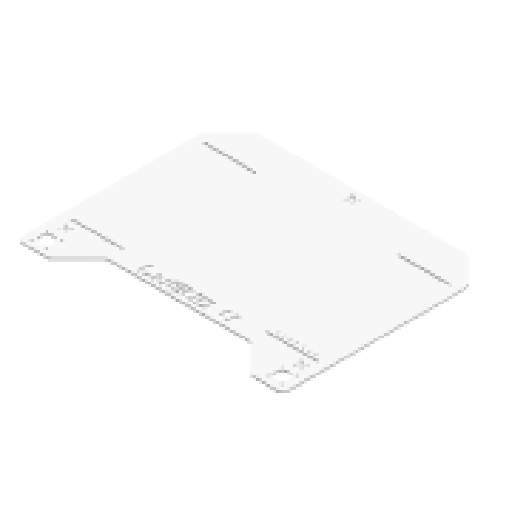
# Autodesk Inventor part: Z Axis Base
Saved by Autodesk Inventor 2023.2 (Build 272271000, 271)
## iProperties
Created: 2023-02-02
Part Number: Z Axis Base
Material: Aluminum 6061
Document SubType Name: Modeling
Designer: remop
Density: 2.7 g/cm^3
Appearance: Aluminum - Dark
Author: remop
Autodesk Inventor part; units mm, degrees
ref_plane "YZ Plane" through (0, 0, 0) normal (1, 0, 0) x (0, 1, 0)
ref_plane "XZ Plane" through (0, 0, 0) normal (0, 1, 0) x (-1, 0, 0)
ref_plane "XY Plane" through (0, 0, 0) normal (0, 0, 1) x (1, 0, 0)
sketch "Sketch1" plane through (0, 0, 0) normal (0, 1, 0) x (-1, 0, 0)
  circle A0 centre (158.2314, 130.3812) radius 11.25 projected
  circle A1 centre (158.2314, 160.3812) radius 6 projected
  circle A2 centre (-213.7686, 130.3812) radius 11.25 projected
  circle A3 centre (-213.7686, 160.3812) radius 6 projected
  circle A4 centre (-27.7686, -135.6188) radius 11 projected
  circle A5 centre (125.7314, 112.8812) radius 1.75
  circle A6 centre (125.7314, -96.1188) radius 1.75
  circle A7 centre (-181.2686, -96.1188) radius 1.75
  circle A8 centre (-181.2686, 112.8812) radius 1.75
  line L0 (222.2314, 188.3812) -> (-277.7686, 188.3812) projected
  line L1 (222.2314, -171.6188) -> (-277.7686, -171.6188) projected
  line L2 (182.2314, 183.3812) -> (132.2314, 183.3812)
  line L3 (132.2314, 183.3812) -> (86.7314, 137.8812)
  line L4 (86.7314, 137.8812) -> (-142.2686, 137.8812)
  line L5 (-142.2686, 137.8812) -> (-187.7686, 183.3812)
  line L6 (-187.7686, 183.3812) -> (-237.7686, 183.3812)
  line L7 (-237.7686, 183.3812) -> (-237.7686, -151.6188)
  line L8 (-237.7686, -151.6188) -> (182.2314, -151.6188)
  line L9 (182.2314, -151.6188) -> (182.2314, 183.3812)
  line L10 (222.2314, -171.6188) -> (222.2314, 188.3812) projected
  line L11 (-277.7686, 188.3812) -> (-277.7686, -171.6188) projected
  circle A9 centre (-213.7686, 160.3812) radius 11.5
  circle A10 centre (-225.2686, 171.8812) radius 2.1
  circle A11 centre (-202.2686, 171.8812) radius 2.1
  circle A12 centre (-202.2686, 148.8812) radius 2.1
  circle A13 centre (-225.2686, 148.8812) radius 2.1
  circle A14 centre (158.2314, 160.3812) radius 11.5
  circle A15 centre (146.7314, 171.8812) radius 2.1
  circle A16 centre (169.7314, 171.8812) radius 2.1
  circle A17 centre (169.7314, 148.8812) radius 2.1
  circle A18 centre (146.7314, 148.8812) radius 2.1
  circle A19 centre (-213.7686, 130.3812) radius 4.5
  circle A20 centre (-219.2686, 124.8812) radius 1.6
  circle A21 centre (-219.2686, 135.8812) radius 1.6
  circle A22 centre (-208.2686, 135.8812) radius 1.6
  circle A23 centre (-208.2686, 124.8812) radius 1.6
  circle A24 centre (158.2314, 130.3812) radius 4.5
  circle A25 centre (152.7314, 135.8812) radius 1.6
  circle A26 centre (163.7314, 135.8812) radius 1.6
  circle A27 centre (163.7314, 124.8812) radius 1.6
  circle A28 centre (152.7314, 124.8812) radius 1.6
  circle A29 centre (-27.7686, -135.6188) radius 4.5
  circle A30 centre (-33.2686, -130.1188) radius 1.6
  circle A31 centre (-22.2686, -130.1188) radius 1.6
  circle A32 centre (-22.2686, -141.1188) radius 1.6
  circle A33 centre (-33.2686, -141.1188) radius 1.6
  point P0 (0, 0)
  point P1 (157.2314, 183.3812)
  dimension "d0" = 307
  dimension "d1" = 209
  dimension "d2" = 3.5
  dimension "d3" = 153.5
  dimension "d4" = 360
  dimension "d5" = 75.5
  dimension "d6" = 5
  dimension "d7" = 40
  dimension "d8" = 20
  dimension "d9" = 40
  dimension "d10" = 5
  dimension "d12" = 45
  dimension "d13" = 50
  dimension "d14" = 45
  dimension "d15" = 25
  dimension "d18" = 23
  dimension "d19" = 11.5
  dimension "d20" = 11.5
  dimension "d21" = 11.5
  dimension "d22" = 11.5
  dimension "d23" = 4.2
  dimension "d24" = 11.5
  dimension "d25" = 11.5
  dimension "d26" = 11.5
  dimension "d27" = 11.5
  dimension "d28" = 9
  dimension "d29" = 5.5
  dimension "d30" = 5.5
  dimension "d31" = 5.5
  dimension "d32" = 5.5
  dimension "d33" = 3.2
  dimension "d35" = 5.5
  dimension "d36" = 5.5
  dimension "d37" = 5.5
  dimension "d39" = 5.5
  dimension "d40" = 5.5
  dimension "d41" = 5.5
  dimension "d42" = 5.5
  dimension "d43" = 5.5
  constraints: 29 centre point, 24 equal radius, 16 end point, 12 horizontal alignment, 12 vertical alignment, 5 coincident, 3 parallel, 1 collinear, 1 horizontal, 1 midpoint, 1 perpendicular
  measures "d0" distance of A8.centre A5.centre
  measures "d1" distance of A6.centre A5.centre
  measures "d2" diameter of A5
  measures "d3" horizontal distance of A6.centre A4.centre
  measures "d4" distance between parallel lines of L1 L0
  measures "d5" distance from line of L1 A7.centre
  measures "d6" distance between parallel lines of L0 L6
  measures "d7" distance between parallel lines of L11 L7
  measures "d8" distance between parallel lines of L1 L8
  measures "d9" distance between parallel lines of L10 L9
  measures "d10" distance from line of L0 point (157.231, 183.381)
  measures "d12" angle of L2 L3
  measures "d13" distance of L2.start L2.end
  measures "d14" angle of L6 L5
  measures "d15" distance from line of A5.centre L4
  measures "d18" diameter of A9
  measures "d19" horizontal distance of A3.centre A10.centre
  measures "d20" horizontal distance of A3.centre A11.centre
  measures "d21" horizontal distance of A10.centre A9.centre
  measures "d22" horizontal distance of A13.centre A3.centre
  measures "d23" diameter of A13
  measures "d24" horizontal distance of A15.centre A1.centre
  measures "d25" horizontal distance of A18.centre A1.centre
  measures "d26" horizontal distance of A1.centre A18.centre
  measures "d27" horizontal distance of A17.centre A14.centre
  measures "d28" diameter of A19
  measures "d29" horizontal distance of A21.centre A2.centre
  measures "d30" horizontal distance of A19.centre A21.centre
  measures "d31" horizontal distance of A22.centre A2.centre
  measures "d32" horizontal distance of A20.centre A2.centre
  measures "d33" diameter of A20
  measures "d35" horizontal distance of A25.centre A0.centre
  measures "d36" horizontal distance of A25.centre A0.centre
  measures "d37" horizontal distance of A0.centre A26.centre
  measures "d39" horizontal distance of A0.centre A28.centre
  measures "d40" horizontal distance of A31.centre A29.centre
  measures "d41" horizontal distance of A30.centre A4.centre
  measures "d42" horizontal distance of A31.centre A29.centre
  measures "d43" horizontal distance of A32.centre A29.centre
extrude "Extrusion1" add sketch "Sketch1" along normal blind 3 contours A0 | A2 | A4 | L9 L8 L7 L6 L5 L4 L3 L2
sketch "Sketch2" plane through (0, 3, 0) normal (0, 1, 0) x (1, 0, 0)
  line L0 (-132.2314, -183.3812) -> (-86.7314, -137.8812) projected
  line L1 (-86.7314, -137.8812) -> (142.2686, -137.8812) projected
  line L2 (142.2686, -137.8812) -> (187.7686, -183.3812) projected
  line L3 (187.7686, -183.3812) -> (237.7686, -183.3812) projected
  line L4 (237.7686, -183.3812) -> (237.7686, 151.6188) projected
  line L5 (237.7686, 151.6188) -> (-182.2314, 151.6188) projected
  line L6 (-182.2314, 151.6188) -> (-182.2314, -183.3812) projected
  line L7 (-182.2314, -183.3812) -> (-132.2314, -183.3812) projected
  circle A0 centre (-158.2314, -130.3812) radius 4.5 projected
  circle A1 centre (-152.7314, -135.8812) radius 1.6 projected
  circle A2 centre (-163.7314, -135.8812) radius 1.6 projected
  circle A3 centre (-163.7314, -124.8812) radius 1.6 projected
  circle A4 centre (-152.7314, -124.8812) radius 1.6 projected
  circle A5 centre (213.7686, -130.3812) radius 4.5 projected
  circle A6 centre (219.2686, -124.8812) radius 1.6 projected
  circle A7 centre (219.2686, -135.8812) radius 1.6 projected
  circle A8 centre (208.2686, -135.8812) radius 1.6 projected
  circle A9 centre (208.2686, -124.8812) radius 1.6 projected
  circle A10 centre (27.7686, 135.6188) radius 4.5 projected
  circle A11 centre (33.2686, 130.1188) radius 1.6 projected
  circle A12 centre (22.2686, 130.1188) radius 1.6 projected
  circle A13 centre (22.2686, 141.1188) radius 1.6 projected
  circle A14 centre (33.2686, 141.1188) radius 1.6 projected
  circle A15 centre (-125.7314, -112.8812) radius 1.75 projected
  circle A16 centre (-125.7314, 96.1188) radius 1.75 projected
  circle A17 centre (181.2686, 96.1188) radius 1.75 projected
  circle A18 centre (181.2686, -112.8812) radius 1.75 projected
  circle A19 centre (-146.7314, -148.8812) radius 2.1 projected
  circle A20 centre (-169.7314, -148.8812) radius 2.1 projected
  circle A21 centre (-169.7314, -171.8812) radius 2.1 projected
  circle A22 centre (-146.7314, -171.8812) radius 2.1 projected
  circle A23 centre (-158.2314, -160.3812) radius 11.5 projected
  circle A24 centre (225.2686, -148.8812) radius 2.1 projected
  circle A25 centre (202.2686, -148.8812) radius 2.1 projected
  circle A26 centre (202.2686, -171.8812) radius 2.1 projected
  circle A27 centre (225.2686, -171.8812) radius 2.1 projected
  circle A28 centre (213.7686, -160.3812) radius 11.5 projected
  line L8 (-71.2064, -116.1262) -> (126.7436, -116.1262) construction
  line L9 (126.7436, -116.1262) -> (126.7436, -129.6362) construction
  line L10 (126.7436, -129.6362) -> (-71.2064, -129.6362) construction
  line L11 (-71.2064, -129.6362) -> (-71.2064, -116.1262) construction
  line L12 (-41.9641, -132.872) -> (-44.5632, -130.2729)
  line L13 (-44.5632, -130.2729) -> (-44.5632, -112.872)
  line L14 (-44.5632, -112.872) -> (-37.5955, -112.872)
  line L15 (-37.5955, -112.872) -> (-37.5955, -132.872)
  line L16 (-37.5955, -132.872) -> (-41.9641, -132.872)
  line L17 (-36.7844, -132.872) -> (-36.7844, -126.9549)
  line L18 (-36.7844, -126.9549) -> (-23.66, -126.9549)
  line L19 (-23.66, -126.9549) -> (-23.66, -132.872)
  line L20 (-23.66, -132.872) -> (-36.7844, -132.872)
  line L21 (-9.3743, -132.8536) -> (-19.3282, -132.8536)
  line L22 (-19.3282, -132.8536) -> (-22.554, -129.6277)
  line L23 (-22.554, -129.6277) -> (-22.554, -118.4388)
  line L24 (-22.554, -118.4388) -> (-15.4941, -118.4388)
  line L25 (-15.4941, -118.4388) -> (-15.4941, -126.9365)
  line L26 (-15.4941, -126.9365) -> (-9.3743, -126.9365)
  line L27 (-9.3743, -126.9365) -> (-9.3743, -132.8536)
  line L28 (-1.5402, -132.8536) -> (-8.6001, -132.8536)
  line L29 (-8.6001, -132.8536) -> (-8.6001, -118.4388)
  line L30 (-8.6001, -118.4388) -> (-1.5402, -118.4388)
  line L31 (-1.5402, -118.4388) -> (-1.5402, -132.8536)
  line L32 (6.5889, -132.872) -> (2.1649, -132.872)
  line L33 (2.1649, -132.872) -> (-0.4342, -130.2729)
  line L34 (-0.4342, -130.2729) -> (-0.4342, -115.4711)
  line L35 (-0.4342, -115.4711) -> (2.1649, -112.872)
  line L36 (2.1649, -112.872) -> (6.5889, -112.872)
  line L37 (6.5889, -112.872) -> (6.5889, -132.872)
  line L38 (20.5797, -119.0471) -> (7.3999, -119.0471)
  line L39 (7.3999, -119.0471) -> (7.3999, -112.872)
  line L40 (7.3999, -112.872) -> (20.5797, -112.872)
  line L41 (20.5797, -112.872) -> (20.5797, -119.0471)
  line L42 (20.5797, -132.872) -> (7.3999, -132.872)
  line L43 (7.3999, -132.872) -> (7.3999, -126.9549)
  line L44 (7.3999, -126.9549) -> (20.5797, -126.9549)
  line L45 (20.5797, -126.9549) -> (20.5797, -132.872)
  line L46 (20.5797, -124.7061) -> (7.3999, -124.7061)
  line L47 (7.3999, -124.7061) -> (7.3999, -119.8582)
  line L48 (7.3999, -119.8582) -> (20.5797, -119.8582)
  line L49 (20.5797, -119.8582) -> (20.5797, -124.7061)
  line L50 (34.8654, -132.8904) -> (28.3216, -132.8904)
  line L51 (28.3216, -132.8904) -> (21.6856, -126.2545)
  line L52 (21.6856, -126.2545) -> (21.6856, -112.872)
  line L53 (21.6856, -112.872) -> (28.7455, -112.872)
  line L54 (28.7455, -112.872) -> (28.7455, -126.5678)
  line L55 (28.7455, -126.5678) -> (34.8654, -126.5678)
  line L56 (34.8654, -126.5678) -> (34.8654, -132.8904)
  line L57 (35.6396, -132.872) -> (35.6396, -112.872)
  line L58 (35.6396, -112.872) -> (42.5889, -112.872)
  line L59 (42.5889, -112.872) -> (42.5889, -126.2176)
  line L60 (42.5889, -126.2176) -> (35.6396, -132.872)
  line L61 (50.7548, -132.872) -> (46.2939, -132.872)
  line L62 (46.2939, -132.872) -> (43.6949, -130.2729)
  line L63 (43.6949, -130.2729) -> (43.6949, -115.4711)
  line L64 (43.6949, -115.4711) -> (46.3124, -112.872)
  line L65 (46.3124, -112.872) -> (56.8746, -112.872)
  line L66 (56.8746, -112.872) -> (56.8746, -119.0471)
  line L67 (56.8746, -119.0471) -> (50.7548, -119.0471)
  line L68 (50.7548, -119.0471) -> (50.7548, -132.872)
  line L69 (64.7087, -130.2545) -> (62.0912, -132.872)
  line L70 (62.0912, -132.872) -> (51.4921, -132.872)
  line L71 (51.4921, -132.872) -> (51.4921, -126.9549)
  line L72 (51.4921, -126.9549) -> (57.6488, -126.9549)
  line L73 (57.6488, -126.9549) -> (57.6488, -112.872)
  line L74 (57.6488, -112.872) -> (62.0912, -112.872)
  line L75 (62.0912, -112.872) -> (64.7087, -115.4895)
  line L76 (64.7087, -115.4895) -> (64.7087, -130.2545)
  line L77 (92.9299, -132.8904) -> (86.3861, -132.8904)
  line L78 (86.3861, -132.8904) -> (79.7502, -126.2545)
  line L79 (79.7502, -126.2545) -> (79.7502, -112.872)
  line L80 (79.7502, -112.872) -> (86.8101, -112.872)
  line L81 (86.8101, -112.872) -> (86.8101, -126.5678)
  line L82 (86.8101, -126.5678) -> (92.9299, -126.5678)
  line L83 (92.9299, -126.5678) -> (92.9299, -132.8904)
  line L84 (93.7041, -132.872) -> (93.7041, -112.872)
  line L85 (93.7041, -112.872) -> (100.6534, -112.872)
  line L86 (100.6534, -112.872) -> (100.6534, -126.2176)
  line L87 (100.6534, -126.2176) -> (93.7041, -132.872)
  point P0 (0, 0)
  point P1 (27.7686, -116.1262)
  point P2 (-71.2064, -122.8812)
  dimension "d44" = 15
  constraints: 2 midpoint, 1 vertical alignment, 2 other
  measures "d44" distance from line of L1 point (-71.206, -122.881)
extrude "Extrusion2" cut sketch "Sketch2" against normal through all contours L12 L13 L14 L15 L16 | L17 L18 L19 L20 | L21 L22 L23 L24 L25 L26 L27 | L28 L29 L30 L31 | L32 L33 L34 L35 L36 L37 | L38 L39 L40 L41 | L42 L43 L44 L45 | L46 L47 L48 L49 | L50 L51 L52 L53 L54 L55 L56 | L57 L58 L59 L60 | L61 L62 L63 L64 L65 L66 L67 L68 | L69 L70 L71 L72 L73 L74 L75 L76 | L77 L78 L79 L80 L81 L82 L83 | L84 L85 L86 L87
sketch "Sketch3" plane through (0, 3, 0) normal (0, 1, 0) x (1, 0, 0)
  line L0 (142.2686, -137.8812) -> (187.7686, -183.3812) projected
  line L1 (237.7686, -183.3812) -> (237.7686, 151.6188) projected
  line L2 (237.7686, 151.6188) -> (-182.2314, 151.6188) projected
  line L3 (-182.2314, 151.6188) -> (-182.2314, -183.3812) projected
  line L4 (-132.2314, -183.3812) -> (-86.7314, -137.8812) projected
  line L5 (-139.805, 151.6188) -> (-182.2314, 109.1924)
  line L6 (-182.2314, 151.6188) -> (-182.2314, -183.3812) projected
  line L7 (237.7686, 109.1924) -> (195.3422, 151.6188)
  point P0 (0, 0)
  dimension "d47" = 60
  constraints: 4 end point, 4 point on line, 2 parallel, 1 perpendicular
  measures "d47" distance of L7.start L7.end
extrude "Extrusion3" cut sketch "Sketch3" against normal through all
fillet "Fillet1" radius 10 10 edges at (-182.2314, 1.5, 183.3812) (-132.2314, 1.5, 183.3812) (237.7686, 1.5, 183.3812) (187.7686, 1.5, 183.3812) (142.2686, 1.5, 137.8812) (237.7686, 1.5, -109.1924) (195.3422, 1.5, -151.6188) (-139.805, 1.5, -151.6188) (-182.2314, 1.5, -109.1924) (-86.7314, 1.5, 137.8812)
sketch "Sketch4" plane through (0, 0, 0) normal (0, -1, 0) x (1, 0, 0)
  circle A0 centre (213.7686, 160.3812) radius 11.5 projected
  circle A1 centre (225.2686, 171.8812) radius 2.1 projected
  circle A2 centre (202.2686, 171.8812) radius 2.1 projected
  circle A3 centre (202.2686, 148.8812) radius 2.1 projected
  circle A4 centre (225.2686, 148.8812) radius 2.1 projected
  circle A5 centre (-158.2314, 160.3812) radius 11.5 projected
  circle A6 centre (-146.7314, 171.8812) radius 2.1 projected
  circle A7 centre (-169.7314, 171.8812) radius 2.1 projected
  circle A8 centre (-169.7314, 148.8812) radius 2.1 projected
  circle A9 centre (-146.7314, 148.8812) radius 2.1 projected
  circle A10 centre (181.2686, 112.8812) radius 1.75 projected
  circle A11 centre (181.2686, -96.1188) radius 1.75 projected
  circle A12 centre (-125.7314, -96.1188) radius 1.75 projected
  circle A13 centre (-125.7314, 112.8812) radius 1.75 projected
  circle A14 centre (33.2686, -141.1188) radius 1.6 projected
  circle A15 centre (22.2686, -141.1188) radius 1.6 projected
  circle A16 centre (22.2686, -130.1188) radius 1.6 projected
  circle A17 centre (33.2686, -130.1188) radius 1.6 projected
  circle A18 centre (27.7686, -135.6188) radius 4.5 projected
  circle A19 centre (208.2686, 124.8812) radius 1.6 projected
  circle A20 centre (208.2686, 135.8812) radius 1.6 projected
  circle A21 centre (219.2686, 135.8812) radius 1.6 projected
  circle A22 centre (219.2686, 124.8812) radius 1.6 projected
  circle A23 centre (213.7686, 130.3812) radius 4.5 projected
  circle A24 centre (-152.7314, 124.8812) radius 1.6 projected
  circle A25 centre (-163.7314, 124.8812) radius 1.6 projected
  circle A26 centre (-163.7314, 135.8812) radius 1.6 projected
  circle A27 centre (-152.7314, 135.8812) radius 1.6 projected
  circle A28 centre (-158.2314, 130.3812) radius 4.5 projected
  arc A29 (-182.2314, -105.0503) -> (-179.3025, -112.1213) centre (-172.2314, -105.0503) ccw projected
  line L0 (-179.3025, -112.1213) -> (-142.7339, -148.6899) projected
  arc A30 (-142.7339, -148.6899) -> (-135.6629, -151.6188) centre (-135.6629, -141.6188) ccw projected
  line L1 (191.2001, -151.6188) -> (-135.6629, -151.6188) projected
  arc A31 (191.2001, -151.6188) -> (198.2711, -148.6899) centre (191.2001, -141.6188) ccw projected
  line L2 (198.2711, -148.6899) -> (234.8397, -112.1213) projected
  arc A32 (234.8397, -112.1213) -> (237.7686, -105.0503) centre (227.7686, -105.0503) ccw projected
  line L3 (237.7686, 173.3812) -> (237.7686, -105.0503) projected
  arc A33 (237.7686, 173.3812) -> (227.7686, 183.3812) centre (227.7686, 173.3812) ccw projected
  line L4 (191.9107, 183.3812) -> (227.7686, 183.3812) projected
  arc A34 (191.9107, 183.3812) -> (184.8397, 180.4523) centre (191.9107, 173.3812) ccw projected
  line L5 (145.1975, 140.8101) -> (184.8397, 180.4523) projected
  arc A35 (138.1265, 137.8812) -> (145.1975, 140.8101) centre (138.1265, 147.8812) ccw projected
  line L6 (-82.5893, 137.8812) -> (138.1265, 137.8812) projected
  arc A36 (-89.6603, 140.8101) -> (-82.5893, 137.8812) centre (-82.5893, 147.8812) ccw projected
  line L7 (-129.3025, 180.4523) -> (-89.6603, 140.8101) projected
  arc A37 (-129.3025, 180.4523) -> (-136.3735, 183.3812) centre (-136.3735, 173.3812) ccw projected
  line L8 (-172.2314, 183.3812) -> (-136.3735, 183.3812) projected
  arc A38 (-172.2314, 183.3812) -> (-182.2314, 173.3812) centre (-172.2314, 173.3812) ccw projected
  line L9 (-182.2314, -105.0503) -> (-182.2314, 173.3812) projected
  line L10 (93.7041, 132.872) -> (100.6534, 126.2176) projected
  line L11 (100.6534, 126.2176) -> (100.6534, 112.872) projected
  line L12 (100.6534, 112.872) -> (93.7041, 112.872) projected
  line L13 (93.7041, 112.872) -> (93.7041, 132.872) projected
  line L14 (64.7087, 130.2545) -> (64.7087, 115.4895) projected
  line L15 (64.7087, 115.4895) -> (62.0912, 112.872) projected
  line L16 (62.0912, 112.872) -> (57.6488, 112.872) projected
  line L17 (57.6488, 112.872) -> (57.6488, 126.9549) projected
  line L18 (57.6488, 126.9549) -> (51.4921, 126.9549) projected
  line L19 (51.4921, 126.9549) -> (51.4921, 132.872) projected
  line L20 (51.4921, 132.872) -> (62.0912, 132.872) projected
  line L21 (62.0912, 132.872) -> (64.7087, 130.2545) projected
  line L22 (35.6396, 132.872) -> (42.5889, 126.2176) projected
  line L23 (42.5889, 126.2176) -> (42.5889, 112.872) projected
  line L24 (42.5889, 112.872) -> (35.6396, 112.872) projected
  line L25 (35.6396, 112.872) -> (35.6396, 132.872) projected
  line L26 (20.5797, 124.7061) -> (20.5797, 119.8582) projected
  line L27 (20.5797, 119.8582) -> (7.3999, 119.8582) projected
  line L28 (7.3999, 119.8582) -> (7.3999, 124.7061) projected
  line L29 (7.3999, 124.7061) -> (20.5797, 124.7061) projected
  line L30 (20.5797, 119.0471) -> (20.5797, 112.872) projected
  line L31 (20.5797, 112.872) -> (7.3999, 112.872) projected
  line L32 (7.3999, 112.872) -> (7.3999, 119.0471) projected
  line L33 (7.3999, 119.0471) -> (20.5797, 119.0471) projected
  line L34 (-1.5402, 132.8536) -> (-1.5402, 118.4388) projected
  line L35 (-1.5402, 118.4388) -> (-8.6001, 118.4388) projected
  line L36 (-8.6001, 118.4388) -> (-8.6001, 132.8536) projected
  line L37 (-8.6001, 132.8536) -> (-1.5402, 132.8536) projected
  line L38 (-36.7844, 132.872) -> (-23.66, 132.872) projected
  line L39 (-23.66, 132.872) -> (-23.66, 126.9549) projected
  line L40 (-23.66, 126.9549) -> (-36.7844, 126.9549) projected
  line L41 (-36.7844, 126.9549) -> (-36.7844, 132.872) projected
  line L42 (-41.9641, 132.872) -> (-37.5955, 132.872) projected
  line L43 (-37.5955, 132.872) -> (-37.5955, 112.872) projected
  line L44 (-37.5955, 112.872) -> (-44.5632, 112.872) projected
  line L45 (-44.5632, 112.872) -> (-44.5632, 130.2729) projected
  line L46 (-44.5632, 130.2729) -> (-41.9641, 132.872) projected
  line L47 (-9.3743, 132.8536) -> (-9.3743, 126.9365) projected
  line L48 (-9.3743, 126.9365) -> (-15.4941, 126.9365) projected
  line L49 (-15.4941, 126.9365) -> (-15.4941, 118.4388) projected
  line L50 (-15.4941, 118.4388) -> (-22.554, 118.4388) projected
  line L51 (-22.554, 118.4388) -> (-22.554, 129.6277) projected
  line L52 (-22.554, 129.6277) -> (-19.3282, 132.8536) projected
  line L53 (-19.3282, 132.8536) -> (-9.3743, 132.8536) projected
  line L54 (6.5889, 132.872) -> (6.5889, 112.872) projected
  line L55 (6.5889, 112.872) -> (2.1649, 112.872) projected
  line L56 (2.1649, 112.872) -> (-0.4342, 115.4711) projected
  line L57 (-0.4342, 115.4711) -> (-0.4342, 130.2729) projected
  line L58 (-0.4342, 130.2729) -> (2.1649, 132.872) projected
  line L59 (2.1649, 132.872) -> (6.5889, 132.872) projected
  line L60 (20.5797, 132.872) -> (20.5797, 126.9549) projected
  line L61 (20.5797, 126.9549) -> (7.3999, 126.9549) projected
  line L62 (7.3999, 126.9549) -> (7.3999, 132.872) projected
  line L63 (7.3999, 132.872) -> (20.5797, 132.872) projected
  line L64 (34.8654, 132.8904) -> (34.8654, 126.5678) projected
  line L65 (34.8654, 126.5678) -> (28.7455, 126.5678) projected
  line L66 (28.7455, 126.5678) -> (28.7455, 112.872) projected
  line L67 (28.7455, 112.872) -> (21.6856, 112.872) projected
  line L68 (21.6856, 112.872) -> (21.6856, 126.2545) projected
  line L69 (21.6856, 126.2545) -> (28.3216, 132.8904) projected
  line L70 (28.3216, 132.8904) -> (34.8654, 132.8904) projected
  line L71 (50.7548, 132.872) -> (50.7548, 119.0471) projected
  line L72 (50.7548, 119.0471) -> (56.8746, 119.0471) projected
  line L73 (56.8746, 119.0471) -> (56.8746, 112.872) projected
  line L74 (56.8746, 112.872) -> (46.3124, 112.872) projected
  line L75 (46.3124, 112.872) -> (43.6949, 115.4711) projected
  line L76 (43.6949, 115.4711) -> (43.6949, 130.2729) projected
  line L77 (43.6949, 130.2729) -> (46.2939, 132.872) projected
  line L78 (46.2939, 132.872) -> (50.7548, 132.872) projected
  line L79 (92.9299, 132.8904) -> (92.9299, 126.5678) projected
  line L80 (92.9299, 126.5678) -> (86.8101, 126.5678) projected
  line L81 (86.8101, 126.5678) -> (86.8101, 112.872) projected
  line L82 (86.8101, 112.872) -> (79.7502, 112.872) projected
  line L83 (79.7502, 112.872) -> (79.7502, 126.2545) projected
  line L84 (79.7502, 126.2545) -> (86.3861, 132.8904) projected
  line L85 (86.3861, 132.8904) -> (92.9299, 132.8904) projected
  line L86 (-85.7314, 112.8812) -> (-165.7314, 112.8812) construction
  line L87 (-85.7314, 111.1312) -> (-165.7314, 111.1312)
  line L88 (-165.7314, 114.6312) -> (-85.7314, 114.6312)
  arc A39 (-85.7314, 111.1312) -> (-85.7314, 114.6312) centre (-85.7314, 112.8812) ccw
  arc A40 (-165.7314, 114.6312) -> (-165.7314, 111.1312) centre (-165.7314, 112.8812) ccw
  line L89 (-165.7314, -96.1188) -> (-85.7314, -96.1188) construction
  circle A41 centre (-125.7314, -96.1188) radius 1.75 projected
  line L90 (-165.7314, -97.8688) -> (-85.7314, -97.8688)
  line L91 (-85.7314, -94.3688) -> (-165.7314, -94.3688)
  arc A42 (-165.7314, -94.3688) -> (-165.7314, -97.8688) centre (-165.7314, -96.1188) ccw
  arc A43 (-85.7314, -97.8688) -> (-85.7314, -94.3688) centre (-85.7314, -96.1188) ccw
  line L92 (221.2686, -96.1188) -> (141.2686, -96.1188) construction
  line L93 (221.2686, -97.8688) -> (141.2686, -97.8688)
  line L94 (141.2686, -94.3688) -> (221.2686, -94.3688)
  arc A44 (221.2686, -97.8688) -> (221.2686, -94.3688) centre (221.2686, -96.1188) ccw
  arc A45 (141.2686, -94.3688) -> (141.2686, -97.8688) centre (141.2686, -96.1188) ccw
  line L95 (221.2686, 112.8812) -> (141.2686, 112.8812) construction
  line L96 (221.2686, 111.1312) -> (141.2686, 111.1312)
  line L97 (141.2686, 114.6312) -> (221.2686, 114.6312)
  arc A46 (221.2686, 111.1312) -> (221.2686, 114.6312) centre (221.2686, 112.8812) ccw
  arc A47 (141.2686, 114.6312) -> (141.2686, 111.1312) centre (141.2686, 112.8812) ccw
  line L98 (210.2686, 107.6312) -> (212.2686, 107.6312)
  line L99 (212.2686, 107.6312) -> (212.2686, 102.6312)
  line L100 (212.2686, 102.6312) -> (210.2686, 102.6312)
  line L101 (210.2686, 102.6312) -> (210.2686, 107.6312)
  line L102 (210.2686, 107.6312) -> (212.2686, 102.6312) construction
  line L103 (212.2686, 107.6312) -> (210.2686, 102.6312) construction
  line L104 (202.2686, 107.6312) -> (202.2686, 102.6312)
  line L105 (202.2686, 102.6312) -> (200.2686, 102.6312)
  line L106 (200.2686, 107.6312) -> (202.2686, 107.6312)
  line L107 (200.2686, 102.6312) -> (200.2686, 107.6312)
  line L108 (200.2686, 107.6312) -> (202.2686, 102.6312) construction
  line L109 (202.2686, 107.6312) -> (200.2686, 102.6312) construction
  line L110 (192.2686, 107.6312) -> (192.2686, 102.6312)
  line L111 (192.2686, 102.6312) -> (190.2686, 102.6312)
  line L112 (190.2686, 107.6312) -> (192.2686, 107.6312)
  line L113 (190.2686, 102.6312) -> (190.2686, 107.6312)
  line L114 (190.2686, 107.6312) -> (192.2686, 102.6312) construction
  line L115 (192.2686, 107.6312) -> (190.2686, 102.6312) construction
  line L116 (182.2686, 107.6312) -> (182.2686, 102.6312)
  line L117 (182.2686, 102.6312) -> (180.2686, 102.6312)
  line L118 (180.2686, 107.6312) -> (182.2686, 107.6312)
  line L119 (180.2686, 102.6312) -> (180.2686, 107.6312)
  line L120 (180.2686, 107.6312) -> (182.2686, 102.6312) construction
  line L121 (182.2686, 107.6312) -> (180.2686, 102.6312) construction
  line L122 (172.2686, 107.6312) -> (172.2686, 102.6312)
  line L123 (172.2686, 102.6312) -> (170.2686, 102.6312)
  line L124 (170.2686, 107.6312) -> (172.2686, 107.6312)
  line L125 (170.2686, 102.6312) -> (170.2686, 107.6312)
  line L126 (170.2686, 107.6312) -> (172.2686, 102.6312) construction
  line L127 (172.2686, 107.6312) -> (170.2686, 102.6312) construction
  line L128 (162.2686, 107.6312) -> (162.2686, 102.6312)
  line L129 (162.2686, 102.6312) -> (160.2686, 102.6312)
  line L130 (160.2686, 107.6312) -> (162.2686, 107.6312)
  line L131 (160.2686, 102.6312) -> (160.2686, 107.6312)
  line L132 (160.2686, 107.6312) -> (162.2686, 102.6312) construction
  line L133 (162.2686, 107.6312) -> (160.2686, 102.6312) construction
  line L134 (152.2686, 107.6312) -> (152.2686, 102.6312)
  line L135 (152.2686, 102.6312) -> (150.2686, 102.6312)
  line L136 (150.2686, 107.6312) -> (152.2686, 107.6312)
  line L137 (150.2686, 102.6312) -> (150.2686, 107.6312)
  line L138 (150.2686, 107.6312) -> (152.2686, 102.6312) construction
  line L139 (152.2686, 107.6312) -> (150.2686, 102.6312) construction
  circle A48 centre (181.2686, 112.8812) radius 1.75 projected
  circle A49 centre (-125.7314, -96.1188) radius 1.75 projected
  point P0 (0, 0)
  point P1 (181.2686, 111.1312)
  point P2 (181.2686, 114.6312)
  point P3 (181.2686, -97.8688)
  point P4 (181.2686, -94.3688)
  point P5 (-125.7314, -94.3688)
  point P6 (-125.7314, -97.8688)
  point P7 (-125.7314, 111.1312)
  point P8 (-125.7314, 114.6312)
  point P9 (211.2686, 105.1312)
  point P10 (201.2686, 105.1312)
  point P11 (191.2686, 105.1312)
  point P12 (181.2686, 105.1312)
  point P13 (171.2686, 105.1312)
  point P14 (161.2686, 105.1312)
  point P15 (151.2686, 105.1312)
  point P16 (181.2686, 105.1312)
  dimension "d51" = 80
  dimension "d54" = 5
  dimension "d55" = 2
  dimension "d58" = 10
  dimension "d63" = 7
  constraints: 116 end point, 20 tangent, 16 point on circle, 8 centre point, 7 midpoint, 7 parallel, 3 equal length, 3 horizontal, 2 point on line, 1 perpendicular, 1 vertical alignment, 66 other
  measures "d51" distance of L94.start L94.end
  measures "d54" distance of L100.end L98.start
  measures "d55" distance of L98.start L98.end
  measures "d58" distance of L98.end L104.start
  measures "d63" distance between parallel lines of L97 L118
extrude "Extrusion4" cut sketch "Sketch4" against normal through all contours A10 L97 A46 L96 | A10 L96 A47 L97 | A11 L94 A44 L93 | A11 L93 A45 L94 | A12 L91 A43 L90 | A12 L90 A42 L91 | A13 L88 A39 L87 | A13 L87 A40 L88 | L98 L99 L100 L101 | L104 L105 L107 L106 | L110 L111 L113 L112 | L116 L117 L119 L118 | L122 L123 L125 L124 | L128 L129 L131 L130 | L134 L135 L137 L136
sketch "Sketch5" plane through (0, 3, 0) normal (0, 1, 0) x (1, 0, 0)
  line L0 (-165.7314, -111.1312) -> (-85.7314, -111.1312) projected
  arc A0 (-85.7314, -114.6312) -> (-85.7314, -111.1312) centre (-85.7314, -112.8812) ccw projected
  line L1 (-85.7314, -114.6312) -> (-165.7314, -114.6312) projected
  arc A1 (-165.7314, -111.1312) -> (-165.7314, -114.6312) centre (-165.7314, -112.8812) ccw projected
  line L2 (-85.7314, 94.3688) -> (-165.7314, 94.3688) projected
  arc A2 (-165.7314, 97.8688) -> (-165.7314, 94.3688) centre (-165.7314, 96.1188) ccw projected
  line L3 (-165.7314, 97.8688) -> (-85.7314, 97.8688) projected
  arc A3 (-85.7314, 94.3688) -> (-85.7314, 97.8688) centre (-85.7314, 96.1188) ccw projected
  line L4 (141.2686, 97.8688) -> (221.2686, 97.8688) projected
  arc A4 (221.2686, 94.3688) -> (221.2686, 97.8688) centre (221.2686, 96.1188) ccw projected
  line L5 (221.2686, 94.3688) -> (141.2686, 94.3688) projected
  arc A5 (141.2686, 97.8688) -> (141.2686, 94.3688) centre (141.2686, 96.1188) ccw projected
  line L6 (141.2686, -111.1312) -> (221.2686, -111.1312) projected
  arc A6 (221.2686, -114.6312) -> (221.2686, -111.1312) centre (221.2686, -112.8812) ccw projected
  line L7 (221.2686, -114.6312) -> (141.2686, -114.6312) projected
  arc A7 (141.2686, -111.1312) -> (141.2686, -114.6312) centre (141.2686, -112.8812) ccw projected
  line L8 (190.2686, -102.6312) -> (192.2686, -102.6312) projected
  line L9 (192.2686, -102.6312) -> (192.2686, -107.6312) projected
  line L10 (192.2686, -107.6312) -> (190.2686, -107.6312) projected
  line L11 (190.2686, -107.6312) -> (190.2686, -102.6312) projected
  line L12 (150.2686, -102.6312) -> (152.2686, -102.6312) projected
  line L13 (152.2686, -102.6312) -> (152.2686, -107.6312) projected
  line L14 (152.2686, -107.6312) -> (150.2686, -107.6312) projected
  line L15 (150.2686, -107.6312) -> (150.2686, -102.6312) projected
  line L16 (180.2686, -102.6312) -> (182.2686, -102.6312) projected
  line L17 (182.2686, -102.6312) -> (182.2686, -107.6312) projected
  line L18 (182.2686, -107.6312) -> (180.2686, -107.6312) projected
  line L19 (180.2686, -107.6312) -> (180.2686, -102.6312) projected
  line L20 (200.2686, -102.6312) -> (202.2686, -102.6312) projected
  line L21 (202.2686, -102.6312) -> (202.2686, -107.6312) projected
  line L22 (202.2686, -107.6312) -> (200.2686, -107.6312) projected
  line L23 (200.2686, -107.6312) -> (200.2686, -102.6312) projected
  line L24 (160.2686, -102.6312) -> (162.2686, -102.6312) projected
  line L25 (162.2686, -102.6312) -> (162.2686, -107.6312) projected
  line L26 (162.2686, -107.6312) -> (160.2686, -107.6312) projected
  line L27 (160.2686, -107.6312) -> (160.2686, -102.6312) projected
  line L28 (170.2686, -102.6312) -> (172.2686, -102.6312) projected
  line L29 (172.2686, -102.6312) -> (172.2686, -107.6312) projected
  line L30 (172.2686, -107.6312) -> (170.2686, -107.6312) projected
  line L31 (170.2686, -107.6312) -> (170.2686, -102.6312) projected
  line L32 (212.2686, -102.6312) -> (212.2686, -107.6312) projected
  line L33 (212.2686, -107.6312) -> (210.2686, -107.6312) projected
  line L34 (210.2686, -107.6312) -> (210.2686, -102.6312) projected
  line L35 (210.2686, -102.6312) -> (212.2686, -102.6312) projected
  arc A8 (-179.3025, 112.1213) -> (-182.2314, 105.0503) centre (-172.2314, 105.0503) ccw projected
  line L36 (-182.2314, 105.0503) -> (-182.2314, -173.3812) projected
  arc A9 (-182.2314, -173.3812) -> (-172.2314, -183.3812) centre (-172.2314, -173.3812) ccw projected
  line L37 (-172.2314, -183.3812) -> (-136.3735, -183.3812) projected
  arc A10 (-136.3735, -183.3812) -> (-129.3025, -180.4523) centre (-136.3735, -173.3812) ccw projected
  line L38 (-129.3025, -180.4523) -> (-89.6603, -140.8101) projected
  arc A11 (-82.5893, -137.8812) -> (-89.6603, -140.8101) centre (-82.5893, -147.8812) ccw projected
  line L39 (-82.5893, -137.8812) -> (138.1265, -137.8812) projected
  arc A12 (145.1975, -140.8101) -> (138.1265, -137.8812) centre (138.1265, -147.8812) ccw projected
  line L40 (145.1975, -140.8101) -> (184.8397, -180.4523) projected
  arc A13 (184.8397, -180.4523) -> (191.9107, -183.3812) centre (191.9107, -173.3812) ccw projected
  line L41 (191.9107, -183.3812) -> (227.7686, -183.3812) projected
  arc A14 (227.7686, -183.3812) -> (237.7686, -173.3812) centre (227.7686, -173.3812) ccw projected
  line L42 (237.7686, -173.3812) -> (237.7686, 105.0503) projected
  arc A15 (237.7686, 105.0503) -> (234.8397, 112.1213) centre (227.7686, 105.0503) ccw projected
  line L43 (234.8397, 112.1213) -> (198.2711, 148.6899) projected
  arc A16 (198.2711, 148.6899) -> (191.2001, 151.6188) centre (191.2001, 141.6188) ccw projected
  line L44 (191.2001, 151.6188) -> (-135.6629, 151.6188) projected
  arc A17 (-135.6629, 151.6188) -> (-142.7339, 148.6899) centre (-135.6629, 141.6188) ccw projected
  line L45 (-142.7339, 148.6899) -> (-179.3025, 112.1213) projected
  line L46 (92.9299, -126.5678) -> (92.9299, -132.8904) projected
  line L47 (92.9299, -132.8904) -> (86.3861, -132.8904) projected
  line L48 (86.3861, -132.8904) -> (79.7502, -126.2545) projected
  line L49 (79.7502, -126.2545) -> (79.7502, -112.872) projected
  line L50 (79.7502, -112.872) -> (86.8101, -112.872) projected
  line L51 (86.8101, -112.872) -> (86.8101, -126.5678) projected
  line L52 (86.8101, -126.5678) -> (92.9299, -126.5678) projected
  line L53 (50.7548, -119.0471) -> (50.7548, -132.872) projected
  line L54 (50.7548, -132.872) -> (46.2939, -132.872) projected
  line L55 (46.2939, -132.872) -> (43.6949, -130.2729) projected
  line L56 (43.6949, -130.2729) -> (43.6949, -115.4711) projected
  line L57 (43.6949, -115.4711) -> (46.3124, -112.872) projected
  line L58 (46.3124, -112.872) -> (56.8746, -112.872) projected
  line L59 (56.8746, -112.872) -> (56.8746, -119.0471) projected
  line L60 (56.8746, -119.0471) -> (50.7548, -119.0471) projected
  line L61 (34.8654, -126.5678) -> (34.8654, -132.8904) projected
  line L62 (34.8654, -132.8904) -> (28.3216, -132.8904) projected
  line L63 (28.3216, -132.8904) -> (21.6856, -126.2545) projected
  line L64 (21.6856, -126.2545) -> (21.6856, -112.872) projected
  line L65 (21.6856, -112.872) -> (28.7455, -112.872) projected
  line L66 (28.7455, -112.872) -> (28.7455, -126.5678) projected
  line L67 (28.7455, -126.5678) -> (34.8654, -126.5678) projected
  line L68 (20.5797, -126.9549) -> (20.5797, -132.872) projected
  line L69 (20.5797, -132.872) -> (7.3999, -132.872) projected
  line L70 (7.3999, -132.872) -> (7.3999, -126.9549) projected
  line L71 (7.3999, -126.9549) -> (20.5797, -126.9549) projected
  line L72 (6.5889, -112.872) -> (6.5889, -132.872) projected
  line L73 (6.5889, -132.872) -> (2.1649, -132.872) projected
  line L74 (2.1649, -132.872) -> (-0.4342, -130.2729) projected
  line L75 (-0.4342, -130.2729) -> (-0.4342, -115.4711) projected
  line L76 (-0.4342, -115.4711) -> (2.1649, -112.872) projected
  line L77 (2.1649, -112.872) -> (6.5889, -112.872) projected
  line L78 (-9.3743, -126.9365) -> (-9.3743, -132.8536) projected
  line L79 (-9.3743, -132.8536) -> (-19.3282, -132.8536) projected
  line L80 (-19.3282, -132.8536) -> (-22.554, -129.6277) projected
  line L81 (-22.554, -129.6277) -> (-22.554, -118.4388) projected
  line L82 (-22.554, -118.4388) -> (-15.4941, -118.4388) projected
  line L83 (-15.4941, -118.4388) -> (-15.4941, -126.9365) projected
  line L84 (-15.4941, -126.9365) -> (-9.3743, -126.9365) projected
  line L85 (-37.5955, -132.872) -> (-41.9641, -132.872) projected
  line L86 (-41.9641, -132.872) -> (-44.5632, -130.2729) projected
  line L87 (-44.5632, -130.2729) -> (-44.5632, -112.872) projected
  line L88 (-44.5632, -112.872) -> (-37.5955, -112.872) projected
  line L89 (-37.5955, -112.872) -> (-37.5955, -132.872) projected
  line L90 (-23.66, -132.872) -> (-36.7844, -132.872) projected
  line L91 (-36.7844, -132.872) -> (-36.7844, -126.9549) projected
  line L92 (-36.7844, -126.9549) -> (-23.66, -126.9549) projected
  line L93 (-23.66, -126.9549) -> (-23.66, -132.872) projected
  line L94 (-1.5402, -118.4388) -> (-1.5402, -132.8536) projected
  line L95 (-1.5402, -132.8536) -> (-8.6001, -132.8536) projected
  line L96 (-8.6001, -132.8536) -> (-8.6001, -118.4388) projected
  line L97 (-8.6001, -118.4388) -> (-1.5402, -118.4388) projected
  line L98 (20.5797, -112.872) -> (20.5797, -119.0471) projected
  line L99 (20.5797, -119.0471) -> (7.3999, -119.0471) projected
  line L100 (7.3999, -119.0471) -> (7.3999, -112.872) projected
  line L101 (7.3999, -112.872) -> (20.5797, -112.872) projected
  line L102 (20.5797, -119.8582) -> (20.5797, -124.7061) projected
  line L103 (20.5797, -124.7061) -> (7.3999, -124.7061) projected
  line L104 (7.3999, -124.7061) -> (7.3999, -119.8582) projected
  line L105 (7.3999, -119.8582) -> (20.5797, -119.8582) projected
  line L106 (42.5889, -126.2176) -> (35.6396, -132.872) projected
  line L107 (35.6396, -132.872) -> (35.6396, -112.872) projected
  line L108 (35.6396, -112.872) -> (42.5889, -112.872) projected
  line L109 (42.5889, -112.872) -> (42.5889, -126.2176) projected
  line L110 (64.7087, -115.4895) -> (64.7087, -130.2545) projected
  line L111 (64.7087, -130.2545) -> (62.0912, -132.872) projected
  line L112 (62.0912, -132.872) -> (51.4921, -132.872) projected
  line L113 (51.4921, -132.872) -> (51.4921, -126.9549) projected
  line L114 (51.4921, -126.9549) -> (57.6488, -126.9549) projected
  line L115 (57.6488, -126.9549) -> (57.6488, -112.872) projected
  line L116 (57.6488, -112.872) -> (62.0912, -112.872) projected
  line L117 (62.0912, -112.872) -> (64.7087, -115.4895) projected
  line L118 (100.6534, -126.2176) -> (93.7041, -132.872) projected
  line L119 (93.7041, -132.872) -> (93.7041, -112.872) projected
  line L120 (93.7041, -112.872) -> (100.6534, -112.872) projected
  line L121 (100.6534, -112.872) -> (100.6534, -126.2176) projected
  circle A18 centre (-158.2314, -130.3812) radius 4.5 projected
  circle A19 centre (-152.7314, -135.8812) radius 1.6 projected
  circle A20 centre (-163.7314, -135.8812) radius 1.6 projected
  circle A21 centre (-163.7314, -124.8812) radius 1.6 projected
  circle A22 centre (-152.7314, -124.8812) radius 1.6 projected
  circle A23 centre (213.7686, -130.3812) radius 4.5 projected
  circle A24 centre (219.2686, -124.8812) radius 1.6 projected
  circle A25 centre (219.2686, -135.8812) radius 1.6 projected
  circle A26 centre (208.2686, -135.8812) radius 1.6 projected
  circle A27 centre (208.2686, -124.8812) radius 1.6 projected
  circle A28 centre (27.7686, 135.6188) radius 4.5 projected
  circle A29 centre (33.2686, 130.1188) radius 1.6 projected
  circle A30 centre (22.2686, 130.1188) radius 1.6 projected
  circle A31 centre (22.2686, 141.1188) radius 1.6 projected
  circle A32 centre (33.2686, 141.1188) radius 1.6 projected
  circle A33 centre (-146.7314, -148.8812) radius 2.1 projected
  circle A34 centre (-169.7314, -148.8812) radius 2.1 projected
  circle A35 centre (-169.7314, -171.8812) radius 2.1 projected
  circle A36 centre (-146.7314, -171.8812) radius 2.1 projected
  circle A37 centre (-158.2314, -160.3812) radius 11.5 projected
  circle A38 centre (225.2686, -148.8812) radius 2.1 projected
  circle A39 centre (202.2686, -148.8812) radius 2.1 projected
  circle A40 centre (202.2686, -171.8812) radius 2.1 projected
  circle A41 centre (225.2686, -171.8812) radius 2.1 projected
  circle A42 centre (213.7686, -160.3812) radius 11.5 projected
  point P0 (0, 0)
  point P1 (168.6686, 74.3688)
  point P2 (192.7686, 74.3688)
  point P3 (192.7686, 49.3688)
  point P4 (170.6686, 49.3688)
  dimension "d64" = 24.1
  dimension "d65" = 25
  dimension "d66" = 45
  dimension "d67" = 20
  constraints: 2 horizontal alignment
  measures "d64" distance of point (192.769, 74.369) point (168.669, 74.369)
  measures "d65" vertical distance of point (170.669, 49.369) point (168.669, 74.369)
  measures "d66" distance from line of L42 point (192.769, 74.369)
  measures "d67" distance from line of L5 point (192.769, 74.369)
hole "Hole1" at (168.6686, 3, -74.3688) at (192.7686, 3, -74.3688) at (192.7686, 3, -49.3688) at (170.6686, 3, -49.3688) direction (0, -1, 0) diameter 3 end through all
equation "\"d3\" = 0.5 * d0"
equation "\"d5\" = 0.5 * d4 - 0.5 * d1"
equation "\"d9\" = d7"
equation "\"d10\" = d6"
equation "\"d14\" = d12"
equation "\"d20\" = d19"
equation "\"d21\" = d19"
equation "\"d22\" = d19"
equation "\"d24\" = d19"
equation "\"d25\" = d24"
equation "\"d26\" = d24"
equation "\"d27\" = d26"
equation "\"d30\" = d29"
equation "\"d31\" = d30"
equation "\"d32\" = d29"
equation "\"d35\" = d29"
equation "\"d36\" = d35"
equation "\"d37\" = d36"
equation "\"d39\" = d35"
equation "\"d40\" = d35"
equation "\"d41\" = d40"
equation "\"d42\" = d40"
equation "\"d43\" = d42"
body "Solid1"
